Autodesk Fusion 360 part; units mm, degrees
note: some values were not read from the file. Set by a fixed rule: which sketch regions a step uses.
(part 7 of 15)
  line L5237 (175.845, -74.1858) -> (176.013, -74.227)
  line L5238 (174.033, -75.1418) -> (174.003, -74.9706)
  line L5239 (161.68, -74.2785) -> (161.84, -74.2105)
  line L5240 (175.752, -75.68) -> (174.752, -75.68)
  line L5241 (158.419, -75.6742) -> (158.251, -75.633)
  line L5242 (175.925, -75.6599) -> (175.752, -75.68)
  line L5243 (161.428, -74.5139) -> (161.541, -74.3815)
  line L5244 (176.301, -74.4185) -> (176.403, -74.5584)
  line L5245 (174.416, -74.2594) -> (174.579, -74.2001)
  line L5246 (174.014, -74.7972) -> (174.064, -74.6309)
  line L5247 (161.302, -74.93) -> (161.308, -74.8373)
  line L5248 (176.471, -74.7182) -> (176.501, -74.8894)
  line L5249 (-22.4283, -74.7218) -> (-22.5199, -74.883)
  line L5250 (159.773, -74.227) -> (159.928, -74.306)
  line L5251 (-23.9795, -74.9953) -> (-24.0947, -74.85)
  line L5252 (-23.1312, -75.2709) -> (-23.3161, -75.2852)
  line L5253 (-22.6221, -73.666) -> (-22.5049, -73.8096)
  line L5254 (-22.3465, -74.3619) -> (-22.3698, -74.5458)
  line L5255 (-23.3161, -75.2852) -> (-23.5002, -75.2632)
  line L5256 (231.239, -72.5669) -> (231.235, -72.6924)
  line L5257 (231.235, -72.6924) -> (231.197, -72.9724)
  line L5258 (231.197, -72.9724) -> (231.12, -73.2443)
  line L5259 (174.003, -74.9706) -> (174.014, -74.7972)
  line L5260 (-22.3698, -74.5458) -> (-22.4283, -74.7218)
  line L5261 (230.857, -73.7424) -> (230.675, -73.9587)
  line L5262 (-23.652, -73.4545) -> (-23.4742, -73.4022)
  line L5263 (-22.7871, -75.1375) -> (-22.9526, -75.2211)
  line L5264 (158.176, -74.2594) -> (158.339, -74.2001)
  line L5265 (231.159, -72.0089) -> (231.219, -72.2851)
  line L5266 (230.675, -73.9587) -> (230.465, -74.1472)
  line L5267 (229.552, -70.5915) -> (229.827, -70.6553)
  line L5268 (231.006, -73.5027) -> (230.857, -73.7424)
  line L5269 (-24.2254, -74.1378) -> (-24.1693, -73.9611)
  line L5270 (-23.8164, -73.5404) -> (-23.652, -73.4545)
  line L5271 (-23.2895, -73.3854) -> (-23.1051, -73.4048)
  line L5272 (-22.3643, -74.1508) -> (-22.3462, -74.3354)
  line L5273 (-22.7649, -73.5478) -> (-22.6221, -73.666)
  line L5274 (230.337, -70.8952) -> (230.561, -71.0666)
  line L5275 (-22.9526, -75.2211) -> (-23.1312, -75.2709)
  line L5276 (-23.4742, -73.4022) -> (-23.2895, -73.3854)
  line L5277 (230.561, -71.0666) -> (230.76, -71.268)
  line L5278 (-23.1051, -73.4048) -> (-22.928, -73.4596)
  line L5279 (229.827, -70.6553) -> (230.09, -70.7572)
  line L5280 (231.219, -72.2851) -> (231.239, -72.5669)
  line L5281 (158.339, -74.2001) -> (158.512, -74.18)
  line L5282 (231.062, -71.7438) -> (231.159, -72.0089)
  line L5283 (230.76, -71.268) -> (230.927, -71.4952)
  line L5284 (-22.4179, -73.9733) -> (-22.3643, -74.1508)
  line L5285 (-22.928, -73.4596) -> (-22.7649, -73.5478)
  line L5286 (-22.3462, -74.3354) -> (-22.3465, -74.3619)
  line L5287 (-23.9609, -73.6566) -> (-23.8164, -73.5404)
  line L5288 (-23.6765, -75.2059) -> (-23.8383, -75.1155)
  line L5289 (231.12, -73.2443) -> (231.006, -73.5027)
  line L5290 (230.09, -70.7572) -> (230.337, -70.8952)
  line L5291 (157.911, -74.4807) -> (158.031, -74.3546)
  line L5292 (158.512, -74.18) -> (159.512, -74.18)
  line L5293 (251.722, -66.4752) -> (251.671, -66.2969)
  line L5294 (-22.5049, -73.8096) -> (-22.4179, -73.9733)
  line L5295 (174.271, -74.3546) -> (174.416, -74.2594)
  line L5296 (157.774, -74.7972) -> (157.824, -74.6309)
  line L5297 (-23.5002, -75.2632) -> (-23.6765, -75.2059)
  line L5298 (-24.0947, -74.85) -> (-24.1795, -74.6851)
  line L5299 (-24.2306, -74.5069) -> (-24.2461, -74.3221)
  line L5300 (-24.1795, -74.6851) -> (-24.2306, -74.5069)
  line L5301 (-24.2461, -74.3221) -> (-24.2254, -74.1378)
  line L5302 (230.927, -71.4952) -> (231.062, -71.7438)
  line L5303 (158.096, -75.554) -> (157.963, -75.4415)
  line L5304 (-22.5199, -74.883) -> (-22.641, -75.0233)
  line L5305 (158.031, -74.3546) -> (158.176, -74.2594)
  line L5306 (-24.08, -73.7986) -> (-23.9609, -73.6566)
  line L5307 (-22.641, -75.0233) -> (-22.7871, -75.1375)
  line L5308 (157.824, -74.6309) -> (157.911, -74.4807)
  line L5309 (-24.1693, -73.9611) -> (-24.08, -73.7986)
  line L5310 (-23.8383, -75.1155) -> (-23.9795, -74.9953)
  line L5311 (159.512, -74.18) -> (159.605, -74.1858)
  line L5312 (158.251, -75.633) -> (158.096, -75.554)
  line L5313 (252.401, -67.0533) -> (252.225, -66.996)
  line L5314 (251.671, -66.2969) -> (251.655, -66.1122)
  line L5315 (253.26, -66.8134) -> (253.114, -66.9276)
  line L5316 (252.085, -65.3305) -> (252.249, -65.2446)
  line L5317 (251.655, -66.1122) -> (251.676, -65.9279)
  line L5318 (251.94, -65.4467) -> (252.085, -65.3305)
  line L5319 (252.585, -67.0752) -> (252.401, -67.0533)
  line L5320 (252.225, -66.996) -> (252.063, -66.9055)
  line L5321 (82.5406, -65.5597) -> (82.6277, -65.7234)
  line L5322 (252.612, -65.1755) -> (252.796, -65.1949)
  line L5323 (253.555, -66.152) -> (253.532, -66.3359)
  line L5324 (252.949, -67.0112) -> (252.77, -67.061)
  line L5325 (252.063, -66.9055) -> (251.922, -66.7854)
  line L5326 (107.112, -72.6524) -> (107.074, -72.9324)
  line L5327 (106.804, -71.4551) -> (106.939, -71.7038)
  line L5328 (106.552, -73.9186) -> (106.342, -74.1071)
  line L5329 (105.852, -74.3863) -> (105.583, -74.4715)
  line L5330 (106.342, -74.1071) -> (106.107, -74.2641)
  line L5331 (105.304, -74.5179) -> (105.022, -74.5246)
  line L5332 (253.114, -66.9276) -> (252.949, -67.0112)
  line L5333 (252.427, -65.1923) -> (252.612, -65.1755)
  line L5334 (106.107, -74.2641) -> (105.852, -74.3863)
  line L5335 (107.074, -72.9324) -> (106.998, -73.2043)
  line L5336 (103.117, -72.464) -> (103.146, -72.1829)
  line L5337 (82.4234, -65.416) -> (82.5406, -65.5597)
  line L5338 (106.637, -71.2279) -> (106.804, -71.4551)
  line L5339 (104.741, -74.4914) -> (104.468, -74.419)
  line L5340 (106.734, -73.7024) -> (106.552, -73.9186)
  line L5341 (105.583, -74.4715) -> (105.304, -74.5179)
  line L5342 (106.883, -73.4626) -> (106.734, -73.7024)
  line L5343 (104.468, -74.419) -> (104.208, -74.3088)
  line L5344 (103.966, -74.1631) -> (103.747, -73.9847)
  line L5345 (103.146, -72.1829) -> (103.214, -71.9088)
  line L5346 (103.214, -71.9088) -> (103.32, -71.6469)
  line L5347 (106.438, -71.0266) -> (106.637, -71.2279)
  line L5348 (107.116, -72.5268) -> (107.112, -72.6524)
  line L5349 (81.9404, -65.1548) -> (82.1175, -65.2096)
  line L5350 (251.807, -66.6401) -> (251.722, -66.4752)
  line L5351 (253.473, -66.5119) -> (253.381, -66.6731)
  line L5352 (82.6277, -65.7234) -> (82.6812, -65.9009)
  line L5353 (252.249, -65.2446) -> (252.427, -65.1923)
  line L5354 (104.208, -74.3088) -> (103.966, -74.1631)
  line L5355 (106.998, -73.2043) -> (106.883, -73.4626)
  line L5356 (103.747, -73.9847) -> (103.555, -73.7773)
  line L5357 (253.555, -66.1255) -> (253.555, -66.152)
  line L5358 (82.1175, -65.2096) -> (82.2806, -65.2978)
  line L5359 (107.036, -71.9688) -> (107.096, -72.245)
  line L5360 (107.096, -72.245) -> (107.116, -72.5268)
  line L5361 (251.732, -65.7512) -> (251.821, -65.5887)
  line L5362 (105.022, -74.5246) -> (104.741, -74.4914)
  line L5363 (103.394, -73.5449) -> (103.268, -73.2922)
  line L5364 (106.939, -71.7038) -> (107.036, -71.9688)
  line L5365 (251.676, -65.9279) -> (251.732, -65.7512)
  line L5366 (103.179, -73.0242) -> (103.128, -72.7463)
  line L5367 (103.268, -73.2922) -> (103.179, -73.0242)
  line L5368 (103.128, -72.7463) -> (103.117, -72.464)
  line L5369 (103.555, -73.7773) -> (103.394, -73.5449)
  line L5370 (253.532, -66.3359) -> (253.473, -66.5119)
  line L5371 (252.77, -67.061) -> (252.585, -67.0752)
  line L5372 (82.2806, -65.2978) -> (82.4234, -65.416)
  line L5373 (251.922, -66.7854) -> (251.807, -66.6401)
  line L5374 (251.821, -65.5887) -> (251.94, -65.4467)
  line L5375 (253.381, -66.6731) -> (253.26, -66.8134)
  line L5376 (104.588, -70.5977) -> (104.865, -70.5426)
  line L5377 (110.65, -72.6213) -> (110.793, -72.7395)
  line L5378 (110.099, -74.3587) -> (109.915, -74.3368)
  line L5379 (110.91, -72.8832) -> (110.997, -73.0469)
  line L5380 (224.032, -74.3768) -> (223.856, -74.3195)
  line L5381 (224.91, -72.7796) -> (225.027, -72.9233)
  line L5382 (223.302, -73.6205) -> (223.286, -73.4357)
  line L5383 (223.694, -74.2291) -> (223.553, -74.1089)
  line L5384 (110.628, -74.211) -> (110.462, -74.2946)
  line L5385 (103.841, -70.9858) -> (104.071, -70.8215)
  line L5386 (223.286, -73.4357) -> (223.307, -73.2515)
  line L5387 (109.576, -74.189) -> (109.435, -74.0688)
  line L5388 (223.856, -74.3195) -> (223.694, -74.2291)
  line L5389 (223.452, -72.9123) -> (223.571, -72.7702)
  line L5390 (223.716, -72.6541) -> (223.88, -72.5682)
  line L5391 (110.487, -72.5332) -> (110.65, -72.6213)
  line L5392 (111.068, -73.4354) -> (111.045, -73.6194)
  line L5393 (224.767, -72.6614) -> (224.91, -72.7796)
  line L5394 (110.986, -73.7953) -> (110.895, -73.9565)
  line L5395 (223.363, -73.0747) -> (223.452, -72.9123)
  line L5396 (109.32, -73.9235) -> (109.235, -73.7586)
  line L5397 (223.307, -73.2515) -> (223.363, -73.0747)
  line L5398 (110.793, -72.7395) -> (110.91, -72.8832)
  line L5399 (224.604, -72.5732) -> (224.767, -72.6614)
  line L5400 (111.051, -73.2244) -> (111.069, -73.4089)
  line L5401 (224.579, -74.3347) -> (224.401, -74.3846)
  line L5402 (110.997, -73.0469) -> (111.051, -73.2244)
  line L5403 (111.045, -73.6194) -> (110.986, -73.7953)
  line L5404 (223.553, -74.1089) -> (223.437, -73.9636)
  line L5405 (224.745, -74.2511) -> (224.579, -74.3347)
  line L5406 (225.012, -73.9966) -> (224.891, -74.1369)
  line L5407 (110.31, -72.4783) -> (110.487, -72.5332)
  line L5408 (110.895, -73.9565) -> (110.774, -74.0969)
  line L5409 (110.462, -74.2946) -> (110.284, -74.3445)
  line L5410 (109.915, -74.3368) -> (109.738, -74.2795)
  line L5411 (223.88, -72.5682) -> (224.058, -72.5158)
  line L5412 (224.891, -74.1369) -> (224.745, -74.2511)
  line L5413 (225.168, -73.2645) -> (225.186, -73.449)
  line L5414 (224.401, -74.3846) -> (224.216, -74.3988)
  line L5415 (105.147, -70.527) -> (105.429, -70.5514)
  line L5416 (103.462, -71.4026) -> (103.637, -71.1808)
  line L5417 (225.104, -73.8354) -> (225.012, -73.9966)
  line L5418 (224.427, -72.5184) -> (224.604, -72.5732)
  line L5419 (104.071, -70.8215) -> (104.321, -70.6913)
  line L5420 (103.637, -71.1808) -> (103.841, -70.9858)
  line L5421 (104.865, -70.5426) -> (105.147, -70.527)
  line L5422 (223.353, -73.7987) -> (223.302, -73.6205)
  line L5423 (104.321, -70.6913) -> (104.588, -70.5977)
  line L5424 (225.162, -73.6595) -> (225.104, -73.8354)
  line L5425 (103.32, -71.6469) -> (103.462, -71.4026)
  line L5426 (225.114, -73.087) -> (225.168, -73.2645)
  line L5427 (224.243, -72.499) -> (224.427, -72.5184)
  line L5428 (224.058, -72.5158) -> (224.243, -72.499)
  line L5429 (110.284, -74.3445) -> (110.099, -74.3587)
  line L5430 (110.774, -74.0969) -> (110.628, -74.211)
  line L5431 (109.738, -74.2795) -> (109.576, -74.189)
  line L5432 (109.435, -74.0688) -> (109.32, -73.9235)
  line L5433 (111.069, -73.4089) -> (111.068, -73.4354)
  line L5434 (223.437, -73.9636) -> (223.353, -73.7987)
  line L5435 (224.216, -74.3988) -> (224.032, -74.3768)
  line L5436 (223.571, -72.7702) -> (223.716, -72.6541)
  line L5437 (225.186, -73.449) -> (225.186, -73.4755)
  line L5438 (225.027, -72.9233) -> (225.114, -73.087)
  line L5439 (225.186, -73.4755) -> (225.162, -73.6595)
  line L5440 (30.6184, -81.0103) -> (30.7629, -80.8941)
  line L5441 (196.183, -80.7235) -> (196.167, -80.5387)
  line L5442 (196.234, -80.9017) -> (196.183, -80.7235)
  line L5443 (197.772, -81.2399) -> (197.626, -81.3541)
  line L5444 (197.985, -80.9384) -> (197.894, -81.0996)
  line L5445 (138.115, -80.1499) -> (138.169, -80.3274)
  line L5446 (197.626, -81.3541) -> (197.461, -81.4377)
  line L5447 (196.319, -81.0666) -> (196.234, -80.9017)
  line L5448 (138.028, -79.9862) -> (138.115, -80.1499)
  line L5449 (196.188, -80.3545) -> (196.244, -80.1777)
  line L5450 (32.151, -82.0755) -> (32.0594, -82.2367)
  line L5451 (138.169, -80.3274) -> (138.187, -80.5119)
  line L5452 (196.434, -81.2119) -> (196.319, -81.0666)
  line L5453 (197.097, -81.5018) -> (196.913, -81.4798)
  line L5454 (196.167, -80.5387) -> (196.188, -80.3545)
  line L5455 (196.333, -80.0153) -> (196.453, -79.8732)
  line L5456 (137.428, -79.5813) -> (137.605, -79.6362)
  line L5457 (31.9382, -82.377) -> (31.7921, -82.4912)
  line L5458 (197.894, -81.0996) -> (197.772, -81.2399)
  line L5459 (136.364, -80.1377) -> (136.453, -79.9752)
  line L5460 (136.572, -79.8332) -> (136.717, -79.717)
  line L5461 (31.2632, -82.6389) -> (31.0791, -82.6169)
  line L5462 (197.124, -79.602) -> (197.308, -79.6214)
  line L5463 (137.892, -81.1999) -> (137.746, -81.314)
  line L5464 (138.187, -80.5384) -> (138.164, -80.7224)
  line L5465 (196.761, -79.6712) -> (196.939, -79.6188)
  line L5466 (196.575, -81.3321) -> (196.434, -81.2119)
  line L5467 (197.461, -81.4377) -> (197.282, -81.4876)
  line L5468 (30.4099, -81.3148) -> (30.4992, -81.1524)
  line L5469 (137.402, -81.4475) -> (137.217, -81.4617)
  line L5470 (136.857, -81.3825) -> (136.695, -81.292)
  line L5471 (30.3487, -81.8606) -> (30.3332, -81.6758)
  line L5472 (138.164, -80.7224) -> (138.105, -80.8983)
  line L5473 (136.453, -79.9752) -> (136.572, -79.8332)
  line L5474 (313.608, -79.1773) -> (313.751, -79.2955)
  line L5475 (313.751, -79.2955) -> (313.868, -79.4391)
  line L5476 (137.581, -81.3976) -> (137.402, -81.4475)
  line L5477 (137.768, -79.7243) -> (137.911, -79.8425)
  line L5478 (137.605, -79.6362) -> (137.768, -79.7243)
  line L5479 (30.7629, -80.8941) -> (30.9272, -80.8082)
  line L5480 (198.044, -80.7625) -> (197.985, -80.9384)
  line L5481 (196.939, -79.6188) -> (197.124, -79.602)
  line L5482 (196.913, -81.4798) -> (196.737, -81.4225)
  line L5483 (137.033, -81.4398) -> (136.857, -81.3825)
  line L5484 (196.453, -79.8732) -> (196.597, -79.7571)
  line L5485 (196.597, -79.7571) -> (196.761, -79.6712)
  line L5486 (197.649, -79.7644) -> (197.791, -79.8826)
  line L5487 (31.7921, -82.4912) -> (31.6266, -82.5748)
  line L5488 (137.911, -79.8425) -> (138.028, -79.9862)
  line L5489 (313.268, -79.0343) -> (313.445, -79.0891)
  line L5490 (137.217, -81.4617) -> (137.033, -81.4398)
  line L5491 (138.105, -80.8983) -> (138.013, -81.0595)
  line L5492 (138.013, -81.0595) -> (137.892, -81.1999)
  line L5493 (138.187, -80.5119) -> (138.187, -80.5384)
  line L5494 (196.244, -80.1777) -> (196.333, -80.0153)
  line L5495 (136.881, -79.6311) -> (137.059, -79.5787)
  line L5496 (31.4481, -82.6246) -> (31.2632, -82.6389)
  line L5497 (30.9272, -80.8082) -> (31.1051, -80.7559)
  line L5498 (196.737, -81.4225) -> (196.575, -81.3321)
  line L5499 (197.485, -79.6762) -> (197.649, -79.7644)
  line L5500 (30.5997, -82.349) -> (30.4845, -82.2037)
  line L5501 (197.282, -81.4876) -> (197.097, -81.5018)
  line L5502 (30.4845, -82.2037) -> (30.3998, -82.0388)
  line L5503 (30.7409, -82.4692) -> (30.5997, -82.349)
  line L5504 (20.4936, -79.3881) -> (20.6128, -79.2461)
  line L5505 (312.279, -80.4795) -> (312.194, -80.3146)
  line L5506 (21.9326, -80.6128) -> (21.7865, -80.7269)
  line L5507 (136.554, -81.1718) -> (136.439, -81.0265)
  line L5508 (312.535, -80.745) -> (312.394, -80.6248)
  line L5509 (312.143, -80.1364) -> (312.127, -79.9516)
  line L5510 (22.0687, -79.3991) -> (22.1558, -79.5628)
  line L5511 (136.308, -80.3144) -> (136.364, -80.1377)
  line L5512 (20.6128, -79.2461) -> (20.7573, -79.1299)
  line L5513 (136.287, -80.4987) -> (136.308, -80.3144)
  line L5514 (137.746, -81.314) -> (137.581, -81.3976)
  line L5515 (313.242, -80.9004) -> (313.057, -80.9147)
  line L5516 (20.8971, -80.7953) -> (20.7353, -80.7049)
  line L5517 (313.421, -80.8506) -> (313.242, -80.9004)
  line L5518 (136.439, -81.0265) -> (136.354, -80.8616)
  line L5519 (314.027, -79.9914) -> (314.003, -80.1753)
  line L5520 (313.586, -80.767) -> (313.421, -80.8506)
  line L5521 (21.7865, -80.7269) -> (21.621, -80.8105)
  line L5522 (312.412, -79.2861) -> (312.557, -79.1699)
  line L5523 (313.732, -80.6528) -> (313.586, -80.767)
  line L5524 (136.303, -80.6834) -> (136.287, -80.4987)
  line L5525 (313.945, -80.3513) -> (313.853, -80.5125)
  line L5526 (312.557, -79.1699) -> (312.721, -79.084)
  line L5527 (1.0553, -76.6139) -> (1.3188, -76.7158)
  line L5528 (136.717, -79.717) -> (136.881, -79.6311)
  line L5529 (137.059, -79.5787) -> (137.244, -79.5619)
  line L5530 (312.899, -79.0317) -> (313.084, -79.0149)
  line L5531 (312.394, -80.6248) -> (312.279, -80.4795)
  line L5532 (21.6456, -79.049) -> (21.8087, -79.1372)
  line L5533 (312.293, -79.4282) -> (312.412, -79.2861)
  line L5534 (22.1558, -79.5628) -> (22.2093, -79.7403)
  line L5535 (312.148, -79.7674) -> (312.204, -79.5906)
  line L5536 (312.697, -80.8354) -> (312.535, -80.745)
  line L5537 (20.3482, -79.7273) -> (20.4043, -79.5506)
  line L5538 (314.027, -79.9649) -> (314.027, -79.9914)
  line L5539 (20.7353, -80.7049) -> (20.5941, -80.5847)
  line L5540 (20.3275, -79.9115) -> (20.3482, -79.7273)
  line L5541 (313.853, -80.5125) -> (313.732, -80.6528)
  line L5542 (136.354, -80.8616) -> (136.303, -80.6834)
  line L5543 (312.194, -80.3146) -> (312.143, -80.1364)
  line L5544 (314.003, -80.1753) -> (313.945, -80.3513)
  line L5545 (21.8087, -79.1372) -> (21.9515, -79.2554)
  line L5546 (21.621, -80.8105) -> (21.4424, -80.8604)
  line L5547 (312.127, -79.9516) -> (312.148, -79.7674)
  line L5548 (21.4685, -78.9942) -> (21.6456, -79.049)
  line L5549 (21.9515, -79.2554) -> (22.0687, -79.3991)
  line L5550 (22.2093, -79.7403) -> (22.2274, -79.9248)
  line L5551 (313.445, -79.0891) -> (313.608, -79.1773)
  line L5552 (313.084, -79.0149) -> (313.268, -79.0343)
  line L5553 (313.955, -79.6029) -> (314.009, -79.7803)
  line L5554 (136.695, -81.292) -> (136.554, -81.1718)
  line L5555 (312.721, -79.084) -> (312.899, -79.0317)
  line L5556 (313.057, -80.9147) -> (312.873, -80.8927)
  line L5557 (22.0537, -80.4724) -> (21.9326, -80.6128)
  line L5558 (313.868, -79.4391) -> (313.955, -79.6029)
  line L5559 (20.4043, -79.5506) -> (20.4936, -79.3881)
  line L5560 (20.3942, -80.2745) -> (20.343, -80.0963)
  line L5561 (137.244, -79.5619) -> (137.428, -79.5813)
  line L5562 (21.0734, -80.8526) -> (20.8971, -80.7953)
  line L5563 (1.3188, -76.7158) -> (1.5653, -76.8539)
  line L5564 (312.873, -80.8927) -> (312.697, -80.8354)
  line L5565 (314.009, -79.7803) -> (314.027, -79.9649)
  line L5566 (312.204, -79.5906) -> (312.293, -79.4282)
  line L5567 (20.4789, -80.4394) -> (20.3942, -80.2745)
  line L5568 (-0.9019, -79.9834) -> (-1.0936, -79.776)
  line L5569 (21.2841, -78.9748) -> (21.4685, -78.9942)
  line L5570 (-1.2542, -79.5436) -> (-1.3805, -79.2909)
  line L5571 (0.9341, -80.4702) -> (0.6555, -80.5166)
  line L5572 (-1.4699, -79.0229) -> (-1.5207, -78.745)
  line L5573 (2.4473, -78.2437) -> (2.4672, -78.5255)
  line L5574 (2.4672, -78.5255) -> (2.4633, -78.6511)
  line L5575 (1.6931, -80.1058) -> (1.4582, -80.2628)
  line L5576 (5.6611, -78.477) -> (5.8382, -78.5319)
  line L5577 (-0.6828, -80.1618) -> (-0.9019, -79.9834)
  line L5578 (-1.5207, -78.745) -> (-1.5318, -78.4627)
  line L5579 (2.2348, -79.4614) -> (2.0853, -79.7011)
  line L5580 (5.8136, -80.2933) -> (5.635, -80.3432)
  line L5581 (21.2575, -80.8746) -> (21.0734, -80.8526)
  line L5582 (1.4582, -80.2628) -> (1.2035, -80.385)
  line L5583 (-1.3805, -79.2909) -> (-1.4699, -79.0229)
  line L5584 (-0.0605, -76.5964) -> (0.2166, -76.5413)
  line L5585 (2.1559, -77.4538) -> (2.29, -77.7025)
  line L5586 (6.3484, -79.0456) -> (6.402, -79.2231)
  line L5587 (-1.0936, -79.776) -> (-1.2542, -79.5436)
  line L5588 (22.2274, -79.9248) -> (22.2271, -79.9513)
  line L5589 (1.5653, -76.8539) -> (1.7899, -77.0253)
  line L5590 (20.343, -80.0963) -> (20.3275, -79.9115)
  line L5591 (0.0925, -80.4901) -> (-0.1806, -80.4177)
  line L5592 (2.3878, -77.9675) -> (2.4473, -78.2437)
  line L5593 (2.349, -79.203) -> (2.2348, -79.4614)
  line L5594 (1.988, -77.2266) -> (2.1559, -77.4538)
  line L5595 (-1.4349, -77.9075) -> (-1.3288, -77.6456)
  line L5596 (5.8382, -78.5319) -> (6.0013, -78.62)
  line L5597 (2.0853, -79.7011) -> (1.9035, -79.9173)
  line L5598 (0.7801, -76.5501) -> (1.0553, -76.6139)
  line L5599 (-0.3271, -76.69) -> (-0.0605, -76.5964)
  line L5600 (6.2464, -79.9552) -> (6.1252, -80.0956)
  line L5601 (5.4502, -80.3574) -> (5.2661, -80.3355)
  line L5602 (4.7867, -80.0676) -> (4.6715, -79.9223)
  line L5603 (6.2613, -78.8819) -> (6.3484, -79.0456)
  line L5604 (-1.5318, -78.4627) -> (-1.503, -78.1816)
  line L5605 (4.9279, -80.1877) -> (4.7867, -80.0676)
  line L5606 (-0.1806, -80.4177) -> (-0.4407, -80.3075)
  line L5607 (1.9035, -79.9173) -> (1.693, -80.1058)
  line L5608 (21.0994, -78.9916) -> (21.2841, -78.9748)
  line L5609 (5.2661, -80.3355) -> (5.0897, -80.2782)
  line L5610 (0.2166, -76.5413) -> (0.4987, -76.5257)
  line L5611 (5.0897, -80.2782) -> (4.9279, -80.1877)
  line L5612 (4.5868, -79.7573) -> (4.5357, -79.5791)
  line L5613 (6.1442, -78.7382) -> (6.2613, -78.8819)
  line L5614 (22.2271, -79.9513) -> (22.2038, -80.1353)
  line L5615 (-1.503, -78.1816) -> (-1.4349, -77.9075)
  line L5616 (2.4257, -78.9311) -> (2.349, -79.203)
  line L5617 (1.2035, -80.385) -> (0.9341, -80.4702)
  line L5618 (22.2038, -80.1353) -> (22.1453, -80.3112)
  line L5619 (20.7573, -79.1299) -> (20.9216, -79.044)
  line L5620 (2.29, -77.7025) -> (2.3878, -77.9675)
  line L5621 (2.4633, -78.6511) -> (2.4257, -78.9311)
  line L5622 (0.6555, -80.5166) -> (0.373, -80.5233)
  line L5623 (0.373, -80.5233) -> (0.0925, -80.4901)
  line L5624 (-0.4407, -80.3075) -> (-0.6828, -80.1618)
  line L5625 (-1.3288, -77.6456) -> (-1.1869, -77.4013)
  line L5626 (6.3379, -79.794) -> (6.2463, -79.9552)
  line L5627 (21.4424, -80.8604) -> (21.2575, -80.8746)
  line L5628 (20.5941, -80.5847) -> (20.4789, -80.4394)
  line L5629 (22.1453, -80.3112) -> (22.0537, -80.4724)
  line L5630 (20.9216, -79.044) -> (21.0994, -78.9916)
  line L5631 (1.7899, -77.0253) -> (1.988, -77.2266)
  line L5632 (212.493, -79.3017) -> (212.311, -79.5179)
  line L5633 (-0.8076, -76.9845) -> (-0.5778, -76.8202)
  line L5634 (5.9791, -80.2097) -> (5.8136, -80.2933)
  line L5635 (210.907, -76.1264) -> (211.188, -76.1507)
  line L5636 (208.938, -78.6235) -> (208.887, -78.3456)
  line L5637 (212.796, -77.5681) -> (212.855, -77.8443)
  line L5638 (4.9499, -78.6127) -> (5.1142, -78.5268)
  line L5639 (209.506, -79.5841) -> (209.314, -79.3766)
  line L5640 (123.792, -76.1107) -> (124.067, -76.1745)
  line L5641 (208.887, -78.3456) -> (208.876, -78.0633)
  line L5642 (-0.5778, -76.8202) -> (-0.3271, -76.69)
  line L5643 (124.577, -76.4144) -> (124.802, -76.5858)
  line L5644 (124.802, -76.5858) -> (125, -76.7872)
  line L5645 (211.188, -76.1507) -> (211.463, -76.2145)
  line L5646 (210.347, -76.197) -> (210.624, -76.1419)
  line L5647 (210.227, -80.0183) -> (209.967, -79.9081)
  line L5648 (124.067, -76.1745) -> (124.331, -76.2764)
  line L5649 (6.4197, -79.4342) -> (6.3964, -79.6181)
  line L5650 (212.564, -77.0545) -> (212.698, -77.3031)
  line L5651 (212.875, -78.1261) -> (212.871, -78.2517)
  line L5652 (4.5202, -79.3944) -> (4.5408, -79.2101)
  line L5653 (4.5408, -79.2101) -> (4.5969, -79.0334)
  line L5654 (124.331, -76.2764) -> (124.577, -76.4144)
  line L5655 (6.402, -79.2231) -> (6.4201, -79.4076)
  line L5656 (212.643, -79.062) -> (212.493, -79.3017)
  line L5657 (5.635, -80.3432) -> (5.4502, -80.3574)
  line L5658 (212.698, -77.3031) -> (212.796, -77.5681)
  line L5659 (209.314, -79.3766) -> (209.154, -79.1442)
  line L5660 (-1.012, -77.1795) -> (-0.8076, -76.9845)
  line L5661 (212.311, -79.5179) -> (212.101, -79.7064)
  line L5662 (4.5969, -79.0334) -> (4.6862, -78.8709)
  line L5663 (-1.1869, -77.4013) -> (-1.012, -77.1795)
  line L5664 (211.866, -79.8634) -> (211.611, -79.9857)
  line L5665 (210.781, -80.1239) -> (210.5, -80.0907)
  line L5666 (4.8054, -78.7289) -> (4.9499, -78.6127)
  line L5667 (209.396, -76.7801) -> (209.6, -76.5851)
  line L5668 (4.6715, -79.9223) -> (4.5868, -79.7573)
  line L5669 (5.1142, -78.5268) -> (5.2921, -78.4745)
  line L5670 (5.4767, -78.4577) -> (5.6611, -78.477)
  line L5671 (211.063, -80.1172) -> (210.781, -80.1239)
  line L5672 (212.396, -76.8272) -> (212.564, -77.0545)
  line L5673 (209.725, -79.7624) -> (209.506, -79.5841)
  line L5674 (212.757, -78.8036) -> (212.643, -79.062)
  line L5675 (4.6862, -78.8709) -> (4.8054, -78.7289)
  line L5676 (6.4201, -79.4076) -> (6.4197, -79.4342)
  line L5677 (209.221, -77.002) -> (209.396, -76.7801)
  line L5678 (211.342, -80.0709) -> (211.063, -80.1172)
  line L5679 (6.1252, -80.0956) -> (5.9791, -80.2097)
  line L5680 (6.0013, -78.62) -> (6.1441, -78.7382)
  line L5681 (0.4987, -76.5257) -> (0.7801, -76.5501)
  line L5682 (212.871, -78.2517) -> (212.834, -78.5317)
  line L5683 (211.973, -76.4545) -> (212.198, -76.6259)
  line L5684 (212.198, -76.6259) -> (212.396, -76.8272)
  line L5685 (6.3964, -79.6181) -> (6.3379, -79.794)
  line L5686 (212.834, -78.5317) -> (212.757, -78.8036)
  line L5687 (211.611, -79.9857) -> (211.342, -80.0709)
  line L5688 (211.727, -76.3165) -> (211.973, -76.4545)
  line L5689 (212.855, -77.8443) -> (212.875, -78.1261)
  line L5690 (212.101, -79.7064) -> (211.866, -79.8634)
  line L5691 (211.463, -76.2145) -> (211.727, -76.3165)
  line L5692 (4.5357, -79.5791) -> (4.5202, -79.3944)
  line L5693 (5.2921, -78.4745) -> (5.4767, -78.4577)
  line L5694 (121.825, -76.9619) -> (122, -76.74)
  line L5695 (209.6, -76.5851) -> (209.83, -76.4208)
  line L5696 (122.329, -79.7224) -> (122.11, -79.544)
  line L5697 (125.361, -78.7635) -> (125.247, -79.0219)
  line L5698 (122, -76.74) -> (122.205, -76.545)
  line L5699 (121.48, -78.0232) -> (121.509, -77.7422)
  line L5700 (122.11, -79.544) -> (121.919, -79.3365)
  line L5701 (124.216, -79.9456) -> (123.946, -80.0308)
  line L5702 (121.683, -77.2062) -> (121.825, -76.9619)
  line L5703 (208.876, -78.0633) -> (208.905, -77.7823)
  line L5704 (122.832, -79.9782) -> (122.571, -79.8681)
  line L5705 (122.205, -76.545) -> (122.434, -76.3808)
  line L5706 (209.079, -77.2462) -> (209.221, -77.002)
  line L5707 (125.475, -78.2116) -> (125.438, -78.4916)
  line L5708 (123.668, -80.0772) -> (123.385, -80.0838)
  line L5709 (122.685, -76.2505) -> (122.952, -76.1569)
  line L5710 (210.081, -76.2906) -> (210.347, -76.197)
  line L5711 (125.438, -78.4916) -> (125.361, -78.7635)
  line L5712 (123.105, -80.0506) -> (122.832, -79.9782)
  line L5713 (125.479, -78.0861) -> (125.475, -78.2116)
  line L5714 (121.919, -79.3365) -> (121.758, -79.1041)
  line L5715 (125.247, -79.0219) -> (125.097, -79.2616)
  line L5716 (123.946, -80.0308) -> (123.668, -80.0772)
  line L5717 (206.664, -78.4825) -> (206.751, -78.6462)
  line L5718 (121.632, -78.8514) -> (121.542, -78.5834)
  line L5719 (124.47, -79.8233) -> (124.216, -79.9456)
  line L5720 (209.83, -76.4208) -> (210.081, -76.2906)
  line L5721 (125.097, -79.2616) -> (124.916, -79.4779)
  line L5722 (206.216, -79.894) -> (206.037, -79.9438)
  line L5723 (125.302, -77.263) -> (125.4, -77.5281)
  line L5724 (124.705, -79.6664) -> (124.47, -79.8233)
  line L5725 (206.649, -79.5559) -> (206.527, -79.6962)
  line L5726 (123.511, -76.0863) -> (123.792, -76.1107)
  line L5727 (206.527, -79.6962) -> (206.381, -79.8104)
  line L5728 (205.492, -79.8788) -> (205.33, -79.7883)
  line L5729 (121.542, -78.5834) -> (121.491, -78.3055)
  line L5730 (124.916, -79.4779) -> (124.705, -79.6664)
  line L5731 (209.027, -78.8915) -> (208.938, -78.6235)
  line L5732 (122.571, -79.8681) -> (122.329, -79.7224)
  line L5733 (122.434, -76.3808) -> (122.685, -76.2505)
  line L5734 (121.491, -78.3055) -> (121.48, -78.0232)
  line L5735 (206.037, -79.9438) -> (205.852, -79.958)
  line L5736 (125.459, -77.8043) -> (125.479, -78.0861)
  line L5737 (121.758, -79.1041) -> (121.632, -78.8514)
  line L5738 (209.154, -79.1442) -> (209.027, -78.8915)
  line L5739 (121.509, -77.7422) -> (121.577, -77.468)
  line L5740 (123.385, -80.0838) -> (123.105, -80.0506)
  line L5741 (206.751, -78.6462) -> (206.804, -78.8237)
  line L5742 (205.189, -79.6682) -> (205.074, -79.5229)
  line L5743 (204.989, -79.358) -> (204.938, -79.1797)
  line L5744 (123.229, -76.1018) -> (123.511, -76.0863)
  line L5745 (121.577, -77.468) -> (121.683, -77.2062)
  line L5746 (205.668, -79.9361) -> (205.492, -79.8788)
  line L5747 (204.999, -78.634) -> (205.088, -78.4715)
  line L5748 (210.5, -80.0907) -> (210.227, -80.0183)
  line L5749 (209.967, -79.9081) -> (209.725, -79.7624)
  line L5750 (125.168, -77.0144) -> (125.302, -77.263)
  line L5751 (208.905, -77.7823) -> (208.973, -77.5081)
  line L5752 (208.973, -77.5081) -> (209.079, -77.2462)
  line L5753 (210.624, -76.1419) -> (210.907, -76.1264)
  line L5754 (125.4, -77.5281) -> (125.459, -77.8043)
  line L5755 (125, -76.7872) -> (125.168, -77.0144)
  line L5756 (205.088, -78.4715) -> (205.208, -78.3295)
  line L5757 (205.074, -79.5229) -> (204.989, -79.358)
  line L5758 (127.553, -78.7707) -> (127.609, -78.5939)
  line L5759 (205.352, -78.2133) -> (205.516, -78.1274)
  line L5760 (129.274, -78.4425) -> (129.361, -78.6062)
  line L5761 (206.063, -78.0777) -> (206.24, -78.1325)
  line L5762 (206.404, -78.2207) -> (206.546, -78.3389)
  line L5763 (205.208, -78.3295) -> (205.352, -78.2133)
  line L5764 (204.922, -78.995) -> (204.943, -78.8107)
  line L5765 (127.532, -78.9549) -> (127.553, -78.7707)
  line L5766 (128.462, -79.918) -> (128.278, -79.896)
  line L5767 (127.548, -79.1397) -> (127.532, -78.9549)
  line L5768 (128.991, -79.7703) -> (128.826, -79.8539)
  line L5769 (127.94, -79.7483) -> (127.799, -79.6281)
  line L5770 (128.826, -79.8539) -> (128.647, -79.9038)
  line L5771 (128.647, -79.9038) -> (128.462, -79.918)
  line L5772 (127.698, -78.4315) -> (127.818, -78.2894)
  line L5773 (205.694, -78.0751) -> (205.879, -78.0583)
  line L5774 (128.85, -78.0924) -> (129.013, -78.1806)
  line L5775 (206.381, -79.8104) -> (206.216, -79.894)
  line L5776 (205.879, -78.0583) -> (206.063, -78.0777)
  line L5777 (129.137, -79.6562) -> (128.991, -79.7703)
  line L5778 (128.278, -79.896) -> (128.102, -79.8387)
  line L5779 (-5.219, -78.3033) -> (-5.3341, -78.158)
  line L5780 (206.74, -79.3947) -> (206.649, -79.5559)
  line L5781 (205.33, -79.7883) -> (205.189, -79.6682)
  line L5782 (204.943, -78.8107) -> (204.999, -78.634)
  line L5783 (205.516, -78.1274) -> (205.694, -78.0751)
  line L5784 (-3.6092, -77.8538) -> (-3.6677, -78.0298)
  line L5785 (-4.1674, -76.7676) -> (-4.0043, -76.8558)
  line L5786 (129.259, -79.5158) -> (129.137, -79.6562)
  line L5787 (128.304, -78.035) -> (128.489, -78.0182)
  line L5788 (129.432, -78.9682) -> (129.432, -78.9947)
  line L5789 (204.938, -79.1797) -> (204.922, -78.995)
  line L5790 (205.852, -79.958) -> (205.668, -79.9361)
  line L5791 (127.599, -79.3179) -> (127.548, -79.1397)
  line L5792 (129.414, -78.7837) -> (129.432, -78.9682)
  line L5793 (-3.5856, -77.6434) -> (-3.5859, -77.6699)
  line L5794 (129.156, -78.2988) -> (129.274, -78.4425)
  line L5795 (129.432, -78.9947) -> (129.409, -79.1787)
  line L5796 (206.799, -79.2187) -> (206.74, -79.3947)
  line L5797 (206.804, -78.8237) -> (206.822, -79.0083)
  line L5798 (127.609, -78.5939) -> (127.698, -78.4315)
  line L5799 (128.102, -79.8387) -> (127.94, -79.7483)
  line L5800 (129.409, -79.1787) -> (129.35, -79.3546)
  line L5801 (129.35, -79.3546) -> (129.259, -79.5158)
  line L5802 (129.361, -78.6062) -> (129.414, -78.7837)
  line L5803 (206.822, -79.0083) -> (206.822, -79.0348)
  line L5804 (128.673, -78.0376) -> (128.85, -78.0924)
  line L5805 (127.799, -79.6281) -> (127.684, -79.4828)
  line L5806 (122.952, -76.1569) -> (123.229, -76.1018)
  line L5807 (127.684, -79.4828) -> (127.599, -79.3179)
  line L5808 (129.013, -78.1806) -> (129.156, -78.2988)
  line L5809 (206.24, -78.1325) -> (206.404, -78.2207)
  line L5810 (206.546, -78.3389) -> (206.664, -78.4825)
  line L5811 (206.822, -79.0348) -> (206.799, -79.2187)
  line L5812 (254.407, -106.52) -> (254.124, -106.527)
  line L5813 (256.1, -105.206) -> (255.986, -105.465)
  line L5814 (253.068, -106.165) -> (252.849, -105.987)
  line L5815 (253.31, -106.311) -> (253.068, -106.165)
  line L5816 (256.139, -103.971) -> (256.198, -104.247)
  line L5817 (252.316, -103.911) -> (252.422, -103.649)
  line L5818 (255.907, -103.457) -> (256.041, -103.706)
  line L5819 (255.541, -103.029) -> (255.739, -103.23)
  line L5820 (255.444, -106.109) -> (255.209, -106.266)
  line L5821 (254.955, -106.388) -> (254.685, -106.474)
  line L5822 (255.655, -105.921) -> (255.444, -106.109)
  line L5823 (256.177, -104.934) -> (256.1, -105.206)
  line L5824 (256.198, -104.247) -> (256.218, -104.529)
  line L5825 (255.739, -103.23) -> (255.907, -103.457)
  line L5826 (253.571, -106.421) -> (253.31, -106.311)
  line L5827 (252.23, -104.748) -> (252.219, -104.466)
  line L5828 (81.4588, -102.988) -> (81.657, -103.19)
  line L5829 (80.9877, -102.679) -> (81.2342, -102.817)
  line L5830 (82.0179, -105.166) -> (81.9037, -105.425)
  line L5831 (80.7242, -102.577) -> (80.9877, -102.679)
  line L5832 (252.564, -103.405) -> (252.739, -103.183)
  line L5833 (82.1362, -104.489) -> (82.1322, -104.614)
  line L5834 (82.1162, -104.207) -> (82.1362, -104.489)
  line L5835 (80.3244, -106.48) -> (80.0419, -106.486)
  line L5836 (254.124, -106.527) -> (253.844, -106.493)
  line L5837 (252.497, -105.547) -> (252.371, -105.294)
  line L5838 (252.422, -103.649) -> (252.564, -103.405)
  line L5839 (81.1271, -106.226) -> (80.8724, -106.348)
  line L5840 (256.214, -104.654) -> (256.177, -104.934)
  line L5841 (81.5724, -105.881) -> (81.362, -106.069)
  line L5842 (80.449, -102.513) -> (80.7242, -102.577)
  line L5843 (80.8724, -106.348) -> (80.6031, -106.433)
  line L5844 (81.8248, -103.417) -> (81.959, -103.666)
  line L5845 (82.0946, -104.894) -> (82.0179, -105.166)
  line L5846 (80.6031, -106.433) -> (80.3244, -106.48)
  line L5847 (255.209, -106.266) -> (254.955, -106.388)
  line L5848 (82.1322, -104.614) -> (82.0946, -104.894)
  line L5849 (81.657, -103.19) -> (81.8248, -103.417)
  line L5850 (81.9037, -105.425) -> (81.7542, -105.664)
  line L5851 (81.362, -106.069) -> (81.1271, -106.226)
  line L5852 (253.424, -102.693) -> (253.691, -102.6)
  line L5853 (81.7542, -105.664) -> (81.5724, -105.881)
  line L5854 (80.0419, -106.486) -> (79.7614, -106.453)
  line L5855 (253.173, -102.823) -> (253.424, -102.693)
  line L5856 (80.1676, -102.489) -> (80.449, -102.513)
  line L5857 (249.407, -104.48) -> (249.584, -104.535)
  line L5858 (82.0567, -103.931) -> (82.1162, -104.207)
  line L5859 (250.094, -105.049) -> (250.147, -105.226)
  line L5860 (79.3419, -102.653) -> (79.6084, -102.56)
  line L5861 (81.959, -103.666) -> (82.0567, -103.931)
  line L5862 (249.89, -104.741) -> (250.007, -104.885)
  line L5863 (249.584, -104.535) -> (249.747, -104.623)
  line L5864 (78.482, -103.365) -> (78.6569, -103.143)
  line L5865 (253.968, -102.545) -> (254.25, -102.529)
  line L5866 (79.4883, -106.381) -> (79.2282, -106.271)
  line L5867 (253.691, -102.6) -> (253.968, -102.545)
  line L5868 (78.1659, -104.145) -> (78.234, -103.871)
  line L5869 (78.7671, -105.947) -> (78.5753, -105.739)
  line L5870 (78.3401, -103.609) -> (78.482, -103.365)
  line L5871 (78.9861, -106.125) -> (78.7671, -105.947)
  line L5872 (249.747, -104.623) -> (249.89, -104.741)
  line L5873 (252.739, -103.183) -> (252.943, -102.988)
  line L5874 (254.25, -102.529) -> (254.531, -102.553)
  line L5875 (78.5753, -105.739) -> (78.4147, -105.507)
  line L5876 (79.7614, -106.453) -> (79.4883, -106.381)
  line L5877 (79.6084, -102.56) -> (79.8855, -102.504)
  line L5878 (81.2342, -102.817) -> (81.4588, -102.988)
  line L5879 (252.943, -102.988) -> (253.173, -102.823)
  line L5880 (79.8855, -102.504) -> (80.1676, -102.489)
  line L5881 (-64.4295, -106.06) -> (-64.4007, -105.779)
  line L5882 (-56.5494, -106.643) -> (-56.4958, -106.82)
  line L5883 (-63.7996, -107.581) -> (-63.9914, -107.373)
  line L5884 (-63.0784, -108.015) -> (-63.3385, -107.905)
  line L5885 (-56.8965, -106.217) -> (-56.7536, -106.335)
  line L5886 (-64.2266, -105.243) -> (-64.0847, -104.999)
  line L5887 (-64.2783, -106.888) -> (-64.3677, -106.62)
  line L5888 (-58.3776, -106.992) -> (-58.3569, -106.807)
  line L5889 (-57.0596, -106.129) -> (-56.8965, -106.217)
  line L5890 (-63.2248, -104.287) -> (-62.9583, -104.194)
  line L5891 (-58.2262, -107.519) -> (-58.311, -107.355)
  line L5892 (-58.311, -107.355) -> (-58.3621, -107.176)
  line L5893 (-62.5247, -108.12) -> (-62.8053, -108.087)
  line L5894 (-63.4755, -104.417) -> (-63.2248, -104.287)
  line L5895 (-57.0842, -107.891) -> (-57.2627, -107.94)
  line L5896 (-56.6364, -106.479) -> (-56.5494, -106.643)
  line L5897 (-61.4396, -107.86) -> (-61.6943, -107.982)
  line L5898 (-62.8053, -108.087) -> (-63.0784, -108.015)
  line L5899 (-61.9636, -108.067) -> (-62.2423, -108.114)
  line L5900 (-56.7536, -106.335) -> (-56.6364, -106.479)
  line L5901 (-63.9914, -107.373) -> (-64.152, -107.141)
  line L5902 (-63.7054, -104.582) -> (-63.4755, -104.417)
  line L5903 (-62.9583, -104.194) -> (-62.6812, -104.138)
  line L5904 (-58.1111, -107.665) -> (-58.2262, -107.519)
  line L5905 (252.281, -105.026) -> (252.23, -104.748)
  line L5906 (254.685, -106.474) -> (254.407, -106.52)
  line L5907 (255.07, -102.719) -> (255.316, -102.857)
  line L5908 (-57.6057, -106.072) -> (-57.4211, -106.055)
  line L5909 (255.986, -105.465) -> (255.836, -105.704)
  line L5910 (-57.9699, -107.785) -> (-58.1111, -107.665)
  line L5911 (256.218, -104.529) -> (256.214, -104.654)
  line L5912 (252.849, -105.987) -> (252.657, -105.779)
  line L5913 (-57.4476, -107.955) -> (-57.6317, -107.933)
  line L5914 (256.041, -103.706) -> (256.139, -103.971)
  line L5915 (255.836, -105.704) -> (255.655, -105.921)
  line L5916 (-56.4777, -107.005) -> (-56.4781, -107.031)
  line L5917 (-58.2116, -106.468) -> (-58.0924, -106.326)
  line L5918 (254.531, -102.553) -> (254.806, -102.617)
  line L5919 (-56.5013, -107.215) -> (-56.5598, -107.391)
  line L5920 (252.657, -105.779) -> (252.497, -105.547)
  line L5921 (-57.7836, -106.124) -> (-57.6057, -106.072)
  line L5922 (252.219, -104.466) -> (252.248, -104.185)
  line L5923 (-56.4781, -107.031) -> (-56.5013, -107.215)
  line L5924 (252.248, -104.185) -> (252.316, -103.911)
  line L5925 (253.844, -106.493) -> (253.571, -106.421)
  line L5926 (-58.0924, -106.326) -> (-57.9479, -106.21)
  line L5927 (-56.6514, -107.552) -> (-56.7726, -107.693)
  line L5928 (-58.3569, -106.807) -> (-58.3009, -106.631)
  line L5929 (-56.9187, -107.807) -> (-57.0842, -107.891)
  line L5930 (-56.5598, -107.391) -> (-56.6514, -107.552)
  line L5931 (-56.7726, -107.693) -> (-56.9187, -107.807)
  line L5932 (254.806, -102.617) -> (255.07, -102.719)
  line L5933 (-57.808, -107.875) -> (-57.9699, -107.785)
  line L5934 (-56.4958, -106.82) -> (-56.4777, -107.005)
  line L5935 (-58.3009, -106.631) -> (-58.2116, -106.468)
  line L5936 (-57.2627, -107.94) -> (-57.4476, -107.955)
  line L5937 (255.316, -102.857) -> (255.541, -103.029)
  line L5938 (-58.3621, -107.176) -> (-58.3776, -106.992)
  line L5939 (-57.6317, -107.933) -> (-57.808, -107.875)
  line L5940 (-57.4211, -106.055) -> (-57.2367, -106.074)
  line L5941 (-57.9479, -106.21) -> (-57.7836, -106.124)
  line L5942 (252.371, -105.294) -> (252.281, -105.026)
  line L5943 (75.2088, -140.938) -> (75.343, -141.187)
  line L5944 (260.866, -140.05) -> (261.147, -140.075)
  line L5945 (73.426, -144.008) -> (73.1454, -143.974)
  line L5946 (259.684, -143.686) -> (259.465, -143.508)
  line L5947 (71.6724, -142.775) -> (71.583, -142.507)
  line L5948 (259.465, -143.508) -> (259.273, -143.3)
  line L5949 (258.864, -141.706) -> (258.932, -141.432)
  line L5950 (72.1511, -143.468) -> (71.9593, -143.26)
  line L5951 (74.8428, -140.51) -> (75.041, -140.711)
  line L5952 (259.355, -140.704) -> (259.559, -140.509)
  line L5953 (259.18, -140.926) -> (259.355, -140.704)
  line L5954 (259.926, -143.832) -> (259.684, -143.686)
  line L5955 (260.04, -140.214) -> (260.307, -140.121)
  line L5956 (74.1082, -140.098) -> (74.3717, -140.2)
  line L5957 (74.2564, -143.869) -> (73.9871, -143.955)
  line L5958 (73.1454, -143.974) -> (72.8723, -143.902)
  line L5959 (72.6122, -143.792) -> (72.3702, -143.646)
  line L5960 (75.5002, -141.728) -> (75.5202, -142.01)
  line L5961 (71.7987, -143.028) -> (71.6724, -142.775)
  line L5962 (75.343, -141.187) -> (75.4408, -141.452)
  line L5963 (71.583, -142.507) -> (71.5322, -142.229)
  line L5964 (74.746, -143.59) -> (74.5111, -143.747)
  line L5965 (75.5162, -142.135) -> (75.4786, -142.415)
  line L5966 (72.3702, -143.646) -> (72.1511, -143.468)
  line L5967 (74.9564, -143.402) -> (74.746, -143.59)
  line L5968 (255.628, -143.86) -> (255.451, -143.803)
  line L5969 (260.74, -144.048) -> (260.46, -144.015)
  line L5970 (75.4408, -141.452) -> (75.5002, -141.728)
  line L5971 (259.113, -143.068) -> (258.987, -142.815)
  line L5972 (258.932, -141.432) -> (259.038, -141.17)
  line L5973 (75.041, -140.711) -> (75.2088, -140.938)
  line L5974 (75.4019, -142.687) -> (75.2877, -142.946)
  line L5975 (72.8723, -143.902) -> (72.6122, -143.792)
  line L5976 (258.987, -142.815) -> (258.897, -142.547)
  line L5977 (73.833, -140.034) -> (74.1082, -140.098)
  line L5978 (261.825, -143.787) -> (261.571, -143.909)
  line L5979 (258.897, -142.547) -> (258.846, -142.269)
  line L5980 (259.559, -140.509) -> (259.789, -140.345)
  line L5981 (259.273, -143.3) -> (259.113, -143.068)
  line L5982 (74.3717, -140.2) -> (74.6182, -140.338)
  line L5983 (73.7084, -144.001) -> (73.426, -144.008)
  line L5984 (261.571, -143.909) -> (261.301, -143.995)
  line L5985 (75.2877, -142.946) -> (75.1382, -143.185)
  line L5986 (260.307, -140.121) -> (260.584, -140.066)
  line L5987 (260.46, -144.015) -> (260.187, -143.942)
  line L5988 (258.846, -142.269) -> (258.835, -141.987)
  line L5989 (259.038, -141.17) -> (259.18, -140.926)
  line L5990 (74.5111, -143.747) -> (74.2564, -143.869)
  line L5991 (71.9593, -143.26) -> (71.7987, -143.028)
  line L5992 (75.1382, -143.185) -> (74.9564, -143.402)
  line L5993 (71.5322, -142.229) -> (71.5212, -141.947)
  line L5994 (71.5212, -141.947) -> (71.5499, -141.666)
  line L5995 (71.5499, -141.666) -> (71.6181, -141.392)
  line L5996 (262.06, -143.63) -> (261.825, -143.787)
  line L5997 (261.301, -143.995) -> (261.023, -144.041)
  line L5998 (74.6182, -140.338) -> (74.8428, -140.51)
  line L5999 (75.4786, -142.415) -> (75.4019, -142.687)
  line L6000 (258.835, -141.987) -> (258.864, -141.706)
  line L6001 (75.5202, -142.01) -> (75.5162, -142.135)
  line L6002 (73.9871, -143.955) -> (73.7084, -144.001)
  line L6003 (261.023, -144.041) -> (260.74, -144.048)
  line L6004 (260.187, -143.942) -> (259.926, -143.832)
  line L6005 (262.271, -143.442) -> (262.06, -143.63)
  line L6006 (255.838, -141.982) -> (256.023, -142.001)
  line L6007 (255.311, -142.137) -> (255.476, -142.051)
  line L6008 (79.4013, -142.53) -> (79.4549, -142.707)
  line L6009 (78.8911, -142.016) -> (79.0542, -142.104)
  line L6010 (255.812, -143.882) -> (255.628, -143.86)
  line L6011 (256.023, -142.001) -> (256.2, -142.056)
  line L6012 (255.451, -143.803) -> (255.289, -143.712)
  line L6013 (256.699, -143.318) -> (256.608, -143.48)
  line L6014 (78.319, -143.82) -> (78.1427, -143.763)
  line L6015 (256.782, -142.932) -> (256.781, -142.959)
  line L6016 (256.2, -142.056) -> (256.363, -142.144)
  line L6017 (79.473, -142.892) -> (79.4726, -142.919)
  line L6018 (256.781, -142.959) -> (256.758, -143.143)
  line L6019 (79.3909, -143.278) -> (79.2993, -143.44)
  line L6020 (78.1427, -143.763) -> (77.9808, -143.672)
  line L6021 (79.2993, -143.44) -> (79.1781, -143.58)
  line L6022 (281.972, -140.711) -> (281.992, -140.993)
  line L6023 (78.8665, -143.778) -> (78.688, -143.828)
  line L6024 (254.958, -142.558) -> (255.048, -142.395)
  line L6025 (256.363, -142.144) -> (256.506, -142.263)
  line L6026 (79.1971, -142.223) -> (79.3143, -142.366)
  line L6027 (78.5031, -143.842) -> (78.319, -143.82)
  line L6028 (78.714, -141.961) -> (78.8911, -142.016)
  line L6029 (72.7259, -140.174) -> (72.9924, -140.081)
  line L6030 (79.1781, -143.58) -> (79.032, -143.694)
  line L6031 (73.2695, -140.026) -> (73.5516, -140.01)
  line L6032 (77.8396, -143.552) -> (77.7244, -143.407)
  line L6033 (256.487, -143.62) -> (256.341, -143.734)
  line L6034 (256.175, -143.818) -> (255.996, -143.868)
  line L6035 (255.996, -143.868) -> (255.812, -143.882)
  line L6036 (256.341, -143.734) -> (256.175, -143.818)
  line L6037 (71.866, -140.886) -> (72.0409, -140.664)
  line L6038 (79.4726, -142.919) -> (79.4494, -143.102)
  line L6039 (256.608, -143.48) -> (256.487, -143.62)
  line L6040 (78.688, -143.828) -> (78.5031, -143.842)
  line L6041 (77.9808, -143.672) -> (77.8396, -143.552)
  line L6042 (255.148, -143.592) -> (255.033, -143.447)
  line L6043 (256.763, -142.748) -> (256.782, -142.932)
  line L6044 (71.6181, -141.392) -> (71.7241, -141.13)
  line L6045 (72.2453, -140.469) -> (72.4752, -140.305)
  line L6046 (79.3143, -142.366) -> (79.4013, -142.53)
  line L6047 (72.9924, -140.081) -> (73.2695, -140.026)
  line L6048 (73.5516, -140.01) -> (73.833, -140.034)
  line L6049 (79.4549, -142.707) -> (79.473, -142.892)
  line L6050 (79.4494, -143.102) -> (79.3909, -143.278)
  line L6051 (256.758, -143.143) -> (256.699, -143.318)
  line L6052 (255.289, -143.712) -> (255.148, -143.592)
  line L6053 (79.032, -143.694) -> (78.8665, -143.778)
  line L6054 (256.71, -142.57) -> (256.763, -142.748)
  line L6055 (71.7241, -141.13) -> (71.866, -140.886)
  line L6056 (254.948, -143.282) -> (254.897, -143.104)
  line L6057 (255.476, -142.051) -> (255.654, -141.999)
  line L6058 (255.048, -142.395) -> (255.167, -142.253)
  line L6059 (255.654, -141.999) -> (255.838, -141.982)
  line L6060 (79.0542, -142.104) -> (79.1971, -142.223)
  line L6061 (254.882, -142.919) -> (254.902, -142.735)
  line L6062 (254.902, -142.735) -> (254.958, -142.558)
  line L6063 (255.033, -143.447) -> (254.948, -143.282)
  line L6064 (72.0409, -140.664) -> (72.2453, -140.469)
  line L6065 (72.4752, -140.305) -> (72.7259, -140.174)
  line L6066 (255.167, -142.253) -> (255.311, -142.137)
  line L6067 (254.897, -143.104) -> (254.882, -142.919)
  line L6068 (256.506, -142.263) -> (256.623, -142.406)
  line L6069 (256.623, -142.406) -> (256.71, -142.57)
  line L6070 (54.9507, -139.042) -> (55.2142, -139.143)
  line L6071 (281.988, -141.119) -> (281.95, -141.399)
  line L6072 (55.8834, -139.654) -> (56.0513, -139.881)
  line L6073 (281.681, -139.922) -> (281.815, -140.17)
  line L6074 (278.144, -141.759) -> (278.055, -141.491)
  line L6075 (278.338, -139.869) -> (278.513, -139.647)
  line L6076 (278.27, -142.011) -> (278.144, -141.759)
  line L6077 (280.459, -142.938) -> (280.18, -142.984)
  line L6078 (279.344, -142.885) -> (279.084, -142.775)
  line L6079 (77.7391, -142.355) -> (77.8583, -142.213)
  line L6080 (281.513, -139.694) -> (281.681, -139.922)
  line L6081 (279.464, -139.064) -> (279.741, -139.009)
  line L6082 (77.5937, -142.694) -> (77.6498, -142.518)
  line L6083 (280.843, -139.184) -> (281.09, -139.322)
  line L6084 (281.428, -142.385) -> (281.218, -142.574)
  line L6085 (78.0028, -142.097) -> (78.1671, -142.011)
  line L6086 (278.623, -142.451) -> (278.431, -142.244)
  line L6087 (280.983, -142.73) -> (280.728, -142.853)
  line L6088 (280.58, -139.082) -> (280.843, -139.184)
  line L6089 (281.95, -141.399) -> (281.874, -141.671)
  line L6090 (278.717, -139.452) -> (278.947, -139.288)
  line L6091 (279.084, -142.775) -> (278.842, -142.63)
  line L6092 (278.055, -141.491) -> (278.004, -141.213)
  line L6093 (277.993, -140.93) -> (278.022, -140.649)
  line L6094 (55.4607, -139.282) -> (55.6852, -139.453)
  line L6095 (278.004, -141.213) -> (277.993, -140.93)
  line L6096 (280.18, -142.984) -> (279.898, -142.991)
  line L6097 (278.09, -140.375) -> (278.196, -140.113)
  line L6098 (77.5886, -143.063) -> (77.5731, -142.879)
  line L6099 (281.815, -140.17) -> (281.912, -140.435)
  line L6100 (280.728, -142.853) -> (280.459, -142.938)
  line L6101 (278.842, -142.63) -> (278.623, -142.451)
  line L6102 (278.431, -142.244) -> (278.27, -142.011)
  line L6103 (278.196, -140.113) -> (278.338, -139.869)
  line L6104 (279.741, -139.009) -> (280.023, -138.993)
  line L6105 (52.5149, -141.719) -> (52.4255, -141.451)
  line L6106 (78.345, -141.959) -> (78.5296, -141.942)
  line L6107 (77.7244, -143.407) -> (77.6397, -143.242)
  line L6108 (56.0513, -139.881) -> (56.1854, -140.13)
  line L6109 (78.5296, -141.942) -> (78.714, -141.961)
  line L6110 (281.09, -139.322) -> (281.315, -139.493)
  line L6111 (281.759, -141.929) -> (281.61, -142.169)
  line L6112 (281.315, -139.493) -> (281.513, -139.694)
  line L6113 (279.898, -142.991) -> (279.617, -142.958)
  line L6114 (281.61, -142.169) -> (281.428, -142.385)
  line L6115 (281.992, -140.993) -> (281.988, -141.119)
  line L6116 (78.1671, -142.011) -> (78.345, -141.959)
  line L6117 (77.6397, -143.242) -> (77.5886, -143.063)
  line L6118 (281.218, -142.574) -> (280.983, -142.73)
  line L6119 (280.305, -139.018) -> (280.58, -139.082)
  line L6120 (279.198, -139.158) -> (279.464, -139.064)
  line L6121 (280.023, -138.993) -> (280.305, -139.018)
  line L6122 (77.6498, -142.518) -> (77.7391, -142.355)
  line L6123 (55.2142, -139.143) -> (55.4607, -139.282)
  line L6124 (281.874, -141.671) -> (281.759, -141.929)
  line L6125 (77.8583, -142.213) -> (78.0028, -142.097)
  line L6126 (278.513, -139.647) -> (278.717, -139.452)
  line L6127 (278.947, -139.288) -> (279.198, -139.158)
  line L6128 (77.5731, -142.879) -> (77.5937, -142.694)
  line L6129 (55.6852, -139.453) -> (55.8834, -139.654)
  line L6130 (54.6755, -138.978) -> (54.9507, -139.042)
  line L6131 (279.617, -142.958) -> (279.344, -142.885)
  line L6132 (278.022, -140.649) -> (278.09, -140.375)